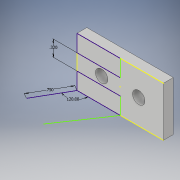
# Autodesk Inventor part: Upper_Spring_Hanger
Saved by Autodesk Inventor 2018.2 (Build 222227000, 227)
## iProperties
Created: 2018-03-24
Part Number: Upper_Spring_Hanger
Material: Generic
Document SubType Name: Modeling
Designer: MIABo
Density: 1 g/cm^3
Appearance: Default
Author: MIABo
Autodesk Inventor part; units mm, degrees
ref_plane "YZ Plane" through (0, 0, 0) normal (1, 0, 0) x (0, 1, 0)
ref_plane "XZ Plane" through (0, 0, 0) normal (0, 1, 0) x (-1, 0, 0)
ref_plane "XY Plane" through (0, 0, 0) normal (0, 0, 1) x (1, 0, 0)
sketch "Sketch1" plane through (0, 0, 0) normal (0, 0, 1) x (1, 0, 0)
  line L0 (-22.225, -12.7) -> (22.225, -12.7)
  line L1 (22.225, -12.7) -> (22.225, 12.7)
  line L2 (22.225, 12.7) -> (-22.225, 12.7)
  line L3 (-22.225, 12.7) -> (-22.225, -12.7)
  line L4 (-22.225, -12.7) -> (22.225, 12.7) construction
  line L5 (22.225, -12.7) -> (-22.225, 12.7) construction
  point P0 (0, 0)
  dimension "d0" = 25.4
  dimension "d1" = 44.45
  constraints: 12 end point, 2 midpoint, 2 parallel, 1 horizontal, 1 perpendicular
  measures "d0" distance of L2.end L0.start
  measures "d1" distance of L1.end L2.end
extrude "Extrusion1" add sketch "Sketch1" along normal blind 5.08
sketch "Sketch2" plane through (0, 0, 5.08) normal (0, 0, 1) x (1, 0, 0)
  line L0 (-22.225, 12.7) -> (-22.225, -12.7) projected
  line L1 (22.225, -12.7) -> (22.225, 12.7) projected
  line L2 (22.225, 12.7) -> (-22.225, 12.7) projected
  point P0 (0, 0)
  point P1 (-9.525, 0)
  point P2 (9.525, 0)
  dimension "d4" = 12.7
  dimension "d5" = 12.7
  dimension "d6" = 12.7
  dimension "d7" = 12.7
  measures "d4" distance from line of L0 point (-9.525, 0)
  measures "d5" distance from line of L1 point (9.525, 0)
  measures "d6" distance from line of L2 point (9.525, 0)
  measures "d7" distance from line of L2 point (-9.525, 0)
hole "Hole1" at (-9.525, 0, 5.08) at (9.525, 0, 5.08) direction (0, 0, -1) diameter 6.35 end through all
sketch "Sketch3" plane through (0, 0, 5.08) normal (0, 0, 1) x (1, 0, 0)
  line L0 (22.225, 12.7) -> (-22.225, 12.7) projected
  line L1 (-22.225, 12.7) -> (0, 12.7)
  line L2 (0, 12.7) -> (0, 4.064)
  line L3 (0, 4.064) -> (-22.225, 4.064)
  line L4 (-22.225, 4.064) -> (-22.225, 12.7)
  line L5 (-22.225, 12.7) -> (-22.225, -12.7) projected
  line L6 (-22.225, -12.7) -> (0, -12.7)
  line L7 (0, -12.7) -> (0, -4.064)
  line L8 (0, -4.064) -> (-22.225, -4.064)
  line L9 (-22.225, -4.064) -> (-22.225, -12.7)
  point P0 (0, 0)
  dimension "d15" = 8.128
  constraints: 16 end point, 4 parallel, 2 horizontal, 2 perpendicular, 1 collinear, 1 point on line
  measures "d15" distance between parallel lines of L3 L8
sketch "Sketch4" plane through (-22.225, -12.7, 0) normal (0, -1, 0) x (1, 0, 0)
  line L0 (0, 5.08) -> (44.45, 5.08) projected
  line L1 (22.225, 5.08) -> (0, 5.08)
  line L2 (0, 5.08) -> (-9.525, 21.5778)
  line L3 (6.35, 28.575) -> (22.225, 5.08)
  point P0 (22.225, 0)
  dimension "d16" = 19.05
  dimension "d17" = 120
  constraints: 6 end point, 1 collinear, 1 midpoint
  measures "d16" distance of L0.start L2.end
  measures "d17" angle of L1 L2
body "Solid1"
